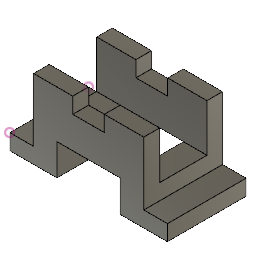
tut 1_P3 (Autodesk Fusion 360 design; units mm, degrees)
Autodesk Fusion 360 part; units mm, degrees
sketch "Sketch1" plane through (0, 0, 0) normal (0, 1, 0) x (1, 0, 0)
  line L0 (0, 0) -> (762, 0)
  line L1 (762, 0) -> (762, -508)
  line L2 (0, 0) -> (0, -254)
  line L3 (0, -254) -> (381, -254)
  line L4 (381, -254) -> (381, -1270)
  line L5 (762, -508) -> (1270, -508)
  line L6 (381, -1270) -> (1016, -1270)
  line L7 (1016, -1270) -> (1016, -1016)
  line L8 (1016, -1016) -> (1270, -1016)
  line L9 (1524, -1016) -> (1270, -1016)
  line L10 (2159, -1270) -> (1524, -1270)
  line L11 (1524, -1270) -> (1524, -1016)
  line L12 (2159, -254) -> (2159, -1270)
  line L13 (2540, -254) -> (2159, -254)
  line L14 (2540, 0) -> (2540, -254)
  line L15 (2540, 0) -> (1778, 0)
  line L16 (1778, 0) -> (1778, -508)
  line L17 (1778, -508) -> (1270, -508)
extrude "Extrude1" add sketch "Sketch1" along normal mid plane 1270
sketch "Sketch2" plane through (0, 0, 254) normal (0, 0, 1) x (-1, 0, 0)
  line L0 (-381, 635) -> (-381, -635)
  line L1 (-381, -635) -> (0, -635)
  line L2 (0, 635) -> (-381, 635)
sketch "Sketch3" plane through (2159, 0, 0) normal (1, 0, 0) x (0, 1, 0)
  line L0 (-635, 254) -> (635, 254)
  line L1 (635, 254) -> (635, 1270)
  line L2 (635, 1270) -> (-635, 1270)
  line L3 (-635, 1270) -> (-635, 254)
  line L4 (-635, 508) -> (635, 508)
  line L5 (-379.7297, 1270) -> (-379.7297, 508)
  line L6 (382.2703, 508) -> (382.2703, 1270)
  line L7 (-379.7297, 1270) -> (382.2703, 1270)
  dimension "d9" = 762
extrude "Extrude2" cut sketch "Sketch3" against normal blind 1778 contours L2 L4 L5 L6 L7
